Autodesk Fusion 360 part; units mm, degrees
(part 6 of 7)
  spline S1643 degree 3 poles (-40.457, 35.67) (-40.4097, 35.6808) (-40.3979, 35.7829) (-40.4495, 35.7797) knots 0 0 0 0 1 1 1 1
  spline S1644 degree 3 poles (-40.4495, 35.7797) (-40.501, 35.7764) (-40.5386, 35.7506) (-40.5773, 35.742) knots 0 0 0 0 1 1 1 1
  spline S1645 degree 3 poles (-40.5773, 35.742) (-40.6235, 35.7334) (-40.674, 35.626) (-40.6096, 35.6302) knots 0 0 0 0 1 1 1 1
  spline S1646 degree 3 poles (-40.5999, 35.2714) (-40.5451, 35.2736) (-40.4989, 35.2983) (-40.457, 35.3068) knots 0 0 0 0 1 1 1 1
  spline S1647 degree 3 poles (-40.457, 35.3068) (-40.414, 35.3176) (-40.4044, 35.4165) (-40.4516, 35.4121) knots 0 0 0 0 1 1 1 1
  spline S1648 degree 3 poles (-40.4516, 35.4121) (-40.4978, 35.4079) (-40.5365, 35.3863) (-40.572, 35.3788) knots 0 0 0 0 1 1 1 1
  spline S1649 degree 3 poles (-40.572, 35.3788) (-40.616, 35.3702) (-40.66, 35.2692) (-40.5999, 35.2714) knots 0 0 0 0 1 1 1 1
  spline S1650 degree 3 poles (-40.5784, 34.8684) (-40.5279, 34.8706) (-40.4828, 34.891) (-40.4441, 34.8996) knots 0 0 0 0 1 1 1 1
  spline S1651 degree 3 poles (-40.4441, 34.8996) (-40.4065, 34.9082) (-40.3958, 35.0006) (-40.4398, 34.9984) knots 0 0 0 0 1 1 1 1
  spline S1652 degree 3 poles (-40.4398, 34.9984) (-40.4839, 34.9941) (-40.5204, 34.9758) (-40.5526, 34.9694) knots 0 0 0 0 1 1 1 1
  spline S1653 degree 3 poles (-40.5526, 34.9694) (-40.5945, 34.963) (-40.6353, 34.8662) (-40.5784, 34.8684) knots 0 0 0 0 1 1 1 1
  spline S1654 degree 3 poles (-40.5118, 34.5664) (-40.4667, 34.5664) (-40.4216, 34.5857) (-40.3872, 34.5932) knots 0 0 0 0 1 1 1 1
  spline S1655 degree 3 poles (-40.3872, 34.5932) (-40.3528, 34.6018) (-40.3431, 34.6835) (-40.384, 34.6835) knots 0 0 0 0 1 1 1 1
  spline S1656 degree 3 poles (-40.384, 34.6835) (-40.4248, 34.6815) (-40.4592, 34.6643) (-40.4903, 34.6588) knots 0 0 0 0 1 1 1 1
  spline S1657 degree 3 poles (-40.4903, 34.6588) (-40.5301, 34.6546) (-40.5633, 34.5644) (-40.5118, 34.5664) knots 0 0 0 0 1 1 1 1
  spline S1658 degree 3 poles (-40.457, 34.1968) (-40.4162, 34.199) (-40.3711, 34.214) (-40.341, 34.2193) knots 0 0 0 0 1 1 1 1
  spline S1659 degree 3 poles (-40.341, 34.2193) (-40.3109, 34.2258) (-40.3023, 34.3009) (-40.3388, 34.3009) knots 0 0 0 0 1 1 1 1
  spline S1660 degree 3 poles (-40.3388, 34.3009) (-40.3764, 34.3009) (-40.4097, 34.2881) (-40.4377, 34.2817) knots 0 0 0 0 1 1 1 1
  spline S1661 degree 3 poles (-40.4377, 34.2817) (-40.4753, 34.2784) (-40.5032, 34.1924) (-40.457, 34.1968) knots 0 0 0 0 1 1 1 1
  spline S1662 degree 3 poles (-40.4022, 33.869) (-40.3646, 33.8712) (-40.3216, 33.8862) (-40.2948, 33.8906) knots 0 0 0 0 1 1 1 1
  spline S1663 degree 3 poles (-40.2948, 33.8906) (-40.269, 33.8948) (-40.2615, 33.9657) (-40.2948, 33.9679) knots 0 0 0 0 1 1 1 1
  spline S1664 degree 3 poles (-40.2948, 33.9679) (-40.3281, 33.97) (-40.3603, 33.9549) (-40.385, 33.9507) knots 0 0 0 0 1 1 1 1
  spline S1665 degree 3 poles (-40.385, 33.9507) (-40.4216, 33.9485) (-40.4441, 33.8668) (-40.4022, 33.869) knots 0 0 0 0 1 1 1 1
  spline S1666 degree 3 poles (-39.9478, 33.6702) (-39.9188, 33.6702) (-39.8747, 33.6788) (-39.8543, 33.681) knots 0 0 0 0 1 1 1 1
  spline S1667 degree 3 poles (-39.8543, 33.681) (-39.8339, 33.6852) (-39.8275, 33.7464) (-39.8565, 33.7475) knots 0 0 0 0 1 1 1 1
  spline S1668 degree 3 poles (-39.8565, 33.7475) (-39.8844, 33.7519) (-39.9156, 33.7411) (-39.936, 33.7411) knots 0 0 0 0 1 1 1 1
  spline S1669 degree 3 poles (-39.936, 33.7411) (-39.9682, 33.7389) (-39.9843, 33.6659) (-39.9478, 33.6702) knots 0 0 0 0 1 1 1 1
  spline S1670 degree 3 poles (-40.992, 35.1521) (-40.961, 35.1546) (-40.9301, 35.159) (-40.8996, 35.1649) knots 0 0 0 0 1 1 1 1
  spline S1671 degree 3 poles (-40.8996, 35.1649) (-40.8781, 35.1693) (-40.8717, 35.2305) (-40.9007, 35.2338) knots 0 0 0 0 1 1 1 1
  spline S1672 degree 3 poles (-40.9007, 35.2338) (-40.9286, 35.2359) (-40.9587, 35.2274) (-40.9802, 35.2252) knots 0 0 0 0 1 1 1 1
  spline S1673 degree 3 poles (-40.9802, 35.2252) (-41.0124, 35.223) (-41.0285, 35.1499) (-40.992, 35.1521) knots 0 0 0 0 1 1 1 1
  spline S1674 degree 3 poles (-39.4998, 33.7519) (-39.4611, 33.7583) (-39.387, 33.7605) (-39.3612, 33.7647) knots 0 0 0 0 1 1 1 1
  spline S1675 degree 3 poles (-39.3612, 33.7647) (-39.3354, 33.7691) (-39.3279, 33.855) (-39.3677, 33.8637) knots 0 0 0 0 1 1 1 1
  spline S1676 degree 3 poles (-39.3677, 33.8637) (-39.4074, 33.8743) (-39.4579, 33.8615) (-39.488, 33.8615) knots 0 0 0 0 1 1 1 1
  spline S1677 degree 3 poles (-39.488, 33.8615) (-39.5395, 33.8604) (-39.5514, 33.7455) (-39.4998, 33.7519) knots 0 0 0 0 1 1 1 1
  spline S1678 degree 3 poles (-39.4772, 33.4499) (-39.4407, 33.4543) (-39.3709, 33.4563) (-39.3462, 33.4607) knots 0 0 0 0 1 1 1 1
  spline S1679 degree 3 poles (-39.3462, 33.4607) (-39.3215, 33.4649) (-39.3139, 33.5466) (-39.3515, 33.5552) knots 0 0 0 0 1 1 1 1
  spline S1680 degree 3 poles (-39.3515, 33.5552) (-39.3891, 33.5659) (-39.4375, 33.5552) (-39.4665, 33.5552) knots 0 0 0 0 1 1 1 1
  spline S1681 degree 3 poles (-39.4665, 33.5552) (-39.5159, 33.5542) (-39.5266, 33.4435) (-39.4772, 33.4499) knots 0 0 0 0 1 1 1 1
  line L717 (-39.4289, 33.0889) -> (-39.3032, 33.0975)
  spline S1682 degree 3 poles (-39.3032, 33.0975) (-39.2796, 33.1017) (-39.272, 33.1792) (-39.3086, 33.1877) knots 0 0 0 0 1 1 1 1
  spline S1683 degree 3 poles (-39.3086, 33.1877) (-39.3451, 33.1985) (-39.3902, 33.1877) (-39.4171, 33.1877) knots 0 0 0 0 1 1 1 1
  spline S1684 degree 3 poles (-39.4171, 33.1877) (-39.4643, 33.1877) (-39.4751, 33.0823) (-39.4289, 33.0889) knots 0 0 0 0 1 1 1 1
  spline S1685 degree 3 poles (-39.373, 32.7299) (-39.3397, 32.7321) (-39.2763, 32.7363) (-39.2538, 32.7407) knots 0 0 0 0 1 1 1 1
  spline S1686 degree 3 poles (-39.2538, 32.7407) (-39.2323, 32.7429) (-39.2248, 32.818) (-39.2591, 32.8245) knots 0 0 0 0 1 1 1 1
  spline S1687 degree 3 poles (-39.2591, 32.8245) (-39.2946, 32.8353) (-39.3365, 32.8245) (-39.3623, 32.8245) knots 0 0 0 0 1 1 1 1
  spline S1688 degree 3 poles (-39.3623, 32.8245) (-39.4074, 32.8245) (-39.4171, 32.7257) (-39.373, 32.7299) knots 0 0 0 0 1 1 1 1
  spline S1689 degree 3 poles (-39.2828, 32.3893) (-39.2516, 32.3936) (-39.1915, 32.3979) (-39.17, 32.4) knots 0 0 0 0 1 1 1 1
  spline S1690 degree 3 poles (-39.17, 32.4) (-39.1496, 32.4043) (-39.1431, 32.4731) (-39.1754, 32.4796) knots 0 0 0 0 1 1 1 1
  spline S1691 degree 3 poles (-39.1754, 32.4796) (-39.2065, 32.4903) (-39.2484, 32.4796) (-39.2731, 32.4796) knots 0 0 0 0 1 1 1 1
  spline S1692 degree 3 poles (-39.2731, 32.4796) (-39.315, 32.4796) (-39.3247, 32.385) (-39.2828, 32.3893) knots 0 0 0 0 1 1 1 1
  line L718 (-39.2258, 32.0186) -> (-39.1206, 32.0271)
  spline S1693 degree 3 poles (-39.1206, 32.0271) (-39.1012, 32.0315) (-39.0948, 32.0959) (-39.1249, 32.1024) knots 0 0 0 0 1 1 1 1
  spline S1694 degree 3 poles (-39.1249, 32.1024) (-39.1549, 32.111) (-39.1936, 32.1024) (-39.2162, 32.1024) knots 0 0 0 0 1 1 1 1
  spline S1695 degree 3 poles (-39.2162, 32.1024) (-39.2559, 32.1024) (-39.2656, 32.0143) (-39.2258, 32.0186) knots 0 0 0 0 1 1 1 1
  line L719 (-39.1216, 31.7037) -> (-39.0239, 31.7101)
  spline S1696 degree 3 poles (-39.0239, 31.7101) (-39.0045, 31.7144) (-39.0002, 31.7757) (-39.0271, 31.7832) knots 0 0 0 0 1 1 1 1
  spline S1697 degree 3 poles (-39.0271, 31.7832) (-39.0561, 31.7897) (-39.0916, 31.7811) (-39.1141, 31.7811) knots 0 0 0 0 1 1 1 1
  spline S1698 degree 3 poles (-39.1141, 31.7811) (-39.1506, 31.7811) (-39.1592, 31.6973) (-39.1216, 31.7037) knots 0 0 0 0 1 1 1 1
  spline S1699 degree 3 poles (-39.0325, 31.3899) (-39.0067, 31.3931) (-38.9573, 31.3953) (-38.9401, 31.3974) knots 0 0 0 0 1 1 1 1
  spline S1700 degree 3 poles (-38.9401, 31.3974) (-38.9229, 31.4007) (-38.9175, 31.4598) (-38.9444, 31.4662) knots 0 0 0 0 1 1 1 1
  spline S1701 degree 3 poles (-38.9444, 31.4662) (-38.9712, 31.4727) (-39.0045, 31.4641) (-39.025, 31.4641) knots 0 0 0 0 1 1 1 1
  spline S1702 degree 3 poles (-39.025, 31.4641) (-39.0593, 31.4641) (-39.0668, 31.3867) (-39.0325, 31.3899) knots 0 0 0 0 1 1 1 1
  spline S1703 degree 3 poles (-39.431, 31.2846) (-39.4074, 31.2889) (-39.358, 31.2911) (-39.3397, 31.2932) knots 0 0 0 0 1 1 1 1
  spline S1704 degree 3 poles (-39.3397, 31.2932) (-39.3236, 31.2964) (-39.3172, 31.3534) (-39.344, 31.3598) knots 0 0 0 0 1 1 1 1
  spline S1705 degree 3 poles (-39.344, 31.3598) (-39.3709, 31.3663) (-39.4042, 31.3577) (-39.4246, 31.3577) knots 0 0 0 0 1 1 1 1
  spline S1706 degree 3 poles (-39.4246, 31.3577) (-39.4579, 31.3577) (-39.4665, 31.2803) (-39.431, 31.2846) knots 0 0 0 0 1 1 1 1
  spline S1707 degree 3 poles (-38.925, 31.0976) (-38.9014, 31.1009) (-38.8552, 31.103) (-38.8402, 31.1051) knots 0 0 0 0 1 1 1 1
  spline S1708 degree 3 poles (-38.8402, 31.1051) (-38.8241, 31.1084) (-38.8187, 31.161) (-38.8434, 31.1675) knots 0 0 0 0 1 1 1 1
  spline S1709 degree 3 poles (-38.8434, 31.1675) (-38.8681, 31.1718) (-38.8993, 31.1643) (-38.9175, 31.1643) knots 0 0 0 0 1 1 1 1
  spline S1710 degree 3 poles (-38.9175, 31.1643) (-38.9498, 31.1643) (-38.9573, 31.0933) (-38.925, 31.0976) knots 0 0 0 0 1 1 1 1
  line L720 (-39.5181, 31.6317) -> (-39.4321, 31.6381)
  spline S1711 degree 3 poles (-39.4321, 31.6381) (-39.4171, 31.6424) (-39.4117, 31.6951) (-39.4364, 31.7015) knots 0 0 0 0 1 1 1 1
  spline S1712 degree 3 poles (-39.4364, 31.7015) (-39.4611, 31.708) (-39.4923, 31.6994) (-39.5116, 31.6994) knots 0 0 0 0 1 1 1 1
  spline S1713 degree 3 poles (-39.5116, 31.6994) (-39.5428, 31.6994) (-39.5503, 31.6274) (-39.5181, 31.6317) knots 0 0 0 0 1 1 1 1
  spline S1714 degree 3 poles (-39.2946, 30.9934) (-39.272, 30.9955) (-39.2258, 30.9977) (-39.2086, 31.0009) knots 0 0 0 0 1 1 1 1
  spline S1715 degree 3 poles (-39.2086, 31.0009) (-39.1936, 31.0031) (-39.1882, 31.0579) (-39.213, 31.0643) knots 0 0 0 0 1 1 1 1
  spline S1716 degree 3 poles (-39.213, 31.0643) (-39.2377, 31.0708) (-39.2688, 31.0632) (-39.2871, 31.0632) knots 0 0 0 0 1 1 1 1
  spline S1717 degree 3 poles (-39.2871, 31.0632) (-39.3193, 31.0622) (-39.3268, 30.9891) (-39.2946, 30.9934) knots 0 0 0 0 1 1 1 1
  line L721 (-38.823, 30.7892) -> (-38.7446, 30.7967)
  spline S1718 degree 3 poles (-38.7446, 30.7967) (-38.7295, 30.7989) (-38.7241, 30.8483) (-38.7478, 30.8537) knots 0 0 0 0 1 1 1 1
  spline S1719 degree 3 poles (-38.7478, 30.8537) (-38.7703, 30.8591) (-38.7983, 30.8526) (-38.8165, 30.8526) knots 0 0 0 0 1 1 1 1
  spline S1720 degree 3 poles (-38.8165, 30.8526) (-38.8455, 30.8515) (-38.852, 30.7849) (-38.823, 30.7892) knots 0 0 0 0 1 1 1 1
  line L722 (-39.575, 32.0014) -> (-39.4966, 32.0078)
  spline S1721 degree 3 poles (-39.4966, 32.0078) (-39.4815, 32.01) (-39.4772, 32.0583) (-39.4998, 32.0648) knots 0 0 0 0 1 1 1 1
  spline S1722 degree 3 poles (-39.4998, 32.0648) (-39.5224, 32.0691) (-39.5514, 32.0626) (-39.5685, 32.0626) knots 0 0 0 0 1 1 1 1
  spline S1723 degree 3 poles (-39.5685, 32.0626) (-39.5986, 32.0626) (-39.6051, 31.9971) (-39.575, 32.0014) knots 0 0 0 0 1 1 1 1
  spline S1724 degree 3 poles (-40.8104, 34.1376) (-40.7879, 34.142) (-40.746, 34.1442) (-40.7309, 34.1462) knots 0 0 0 0 1 1 1 1
  spline S1725 degree 3 poles (-40.7309, 34.1462) (-40.7159, 34.1484) (-40.7116, 34.199) (-40.7342, 34.2054) knots 0 0 0 0 1 1 1 1
  spline S1726 degree 3 poles (-40.7342, 34.2054) (-40.7578, 34.2096) (-40.7857, 34.2032) (-40.8029, 34.2032) knots 0 0 0 0 1 1 1 1
  spline S1727 degree 3 poles (-40.8029, 34.2032) (-40.833, 34.2032) (-40.8395, 34.1356) (-40.8104, 34.1376) knots 0 0 0 0 1 1 1 1
  line L723 (-39.9113, 33.322) -> (-39.8317, 33.3284)
  spline S1728 degree 3 poles (-39.8317, 33.3284) (-39.8178, 33.3306) (-39.8124, 33.379) (-39.835, 33.3854) knots 0 0 0 0 1 1 1 1
  spline S1729 degree 3 poles (-39.835, 33.3854) (-39.8586, 33.3918) (-39.8865, 33.3854) (-39.9048, 33.3854) knots 0 0 0 0 1 1 1 1
  spline S1730 degree 3 poles (-39.9048, 33.3854) (-39.9338, 33.3843) (-39.9413, 33.3178) (-39.9113, 33.322) knots 0 0 0 0 1 1 1 1
  line L724 (-40.9415, 34.8094) -> (-40.8609, 34.8158)
  spline S1731 degree 3 poles (-40.8609, 34.8158) (-40.847, 34.8179) (-40.8427, 34.8684) (-40.8652, 34.8748) knots 0 0 0 0 1 1 1 1
  spline S1732 degree 3 poles (-40.8652, 34.8748) (-40.8878, 34.8791) (-40.9168, 34.8727) (-40.934, 34.8727) knots 0 0 0 0 1 1 1 1
  spline S1733 degree 3 poles (-40.934, 34.8727) (-40.9641, 34.8727) (-40.9705, 34.805) (-40.9415, 34.8094) knots 0 0 0 0 1 1 1 1
  line L725 (-39.2054, 30.7033) -> (-39.127, 30.7097)
  spline S1734 degree 3 poles (-39.127, 30.7097) (-39.113, 30.7119) (-39.1077, 30.7602) (-39.1302, 30.7666) knots 0 0 0 0 1 1 1 1
  spline S1735 degree 3 poles (-39.1302, 30.7666) (-39.1539, 30.772) (-39.1818, 30.7656) (-39.2001, 30.7656) knots 0 0 0 0 1 1 1 1
  spline S1736 degree 3 poles (-39.2001, 30.7656) (-39.2291, 30.7645) (-39.2366, 30.699) (-39.2054, 30.7033) knots 0 0 0 0 1 1 1 1
  spline S1737 degree 3 poles (-40.6729, 33.4768) (-40.6504, 33.4811) (-40.6085, 33.4832) (-40.5924, 33.4854) knots 0 0 0 0 1 1 1 1
  spline S1738 degree 3 poles (-40.5924, 33.4854) (-40.5784, 33.4875) (-40.5741, 33.538) (-40.5967, 33.5424) knots 0 0 0 0 1 1 1 1
  spline S1739 degree 3 poles (-40.5967, 33.5424) (-40.6192, 33.5466) (-40.6482, 33.5402) (-40.6654, 33.5402) knots 0 0 0 0 1 1 1 1
  spline S1740 degree 3 poles (-40.6654, 33.5402) (-40.6955, 33.5402) (-40.7019, 33.4746) (-40.6729, 33.4768) knots 0 0 0 0 1 1 1 1
  line L726 (-40.5483, 32.8288) -> (-40.471, 32.8353)
  spline S1741 degree 3 poles (-40.471, 32.8353) (-40.457, 32.8373) (-40.4505, 32.8879) (-40.4731, 32.8943) knots 0 0 0 0 1 1 1 1
  spline S1742 degree 3 poles (-40.4731, 32.8943) (-40.4968, 32.9007) (-40.5247, 32.8922) (-40.5429, 32.8922) knots 0 0 0 0 1 1 1 1
  spline S1743 degree 3 poles (-40.5429, 32.8922) (-40.572, 32.8911) (-40.5795, 32.8245) (-40.5483, 32.8288) knots 0 0 0 0 1 1 1 1
  line L727 (-38.7123, 30.4679) -> (-38.6414, 30.4744)
  spline S1744 degree 3 poles (-38.6414, 30.4744) (-38.6275, 30.4765) (-38.6232, 30.5217) (-38.6446, 30.527) knots 0 0 0 0 1 1 1 1
  spline S1745 degree 3 poles (-38.6446, 30.527) (-38.6651, 30.5324) (-38.6919, 30.5259) (-38.708, 30.5259) knots 0 0 0 0 1 1 1 1
  spline S1746 degree 3 poles (-38.708, 30.5259) (-38.7338, 30.5259) (-38.7403, 30.4647) (-38.7123, 30.4679) knots 0 0 0 0 1 1 1 1
  spline S1747 degree 3 poles (-40.0047, 36.2202) (-39.966, 36.2309) (-39.9424, 36.2954) (-39.9596, 36.2954) knots 0 0 0 0 1 1 1 1
  spline S1748 degree 3 poles (-39.9596, 36.2954) (-39.9725, 36.2976) (-40.0079, 36.3223) (-40.0552, 36.3126) knots 0 0 0 0 1 1 1 1
  spline S1749 degree 3 poles (-40.0552, 36.3126) (-40.0982, 36.304) (-40.1369, 36.2375) (-40.1089, 36.2353) knots 0 0 0 0 1 1 1 1
  spline S1750 degree 3 poles (-40.1089, 36.2353) (-40.0982, 36.2287) (-40.0552, 36.201) (-40.0047, 36.2202) knots 0 0 0 0 1 1 1 1
  spline S1751 degree 3 poles (-39.9306, 36.6855) (-39.908, 36.6984) (-39.8758, 36.7048) (-39.8489, 36.7145) knots 0 0 0 0 1 1 1 1
  spline S1752 degree 3 poles (-39.8489, 36.7145) (-39.8167, 36.7253) (-39.8135, 36.8048) (-39.864, 36.7962) knots 0 0 0 0 1 1 1 1
  spline S1753 degree 3 poles (-39.864, 36.7962) (-39.8951, 36.7898) (-39.9102, 36.7746) (-39.9306, 36.7693) knots 0 0 0 0 1 1 1 1
  spline S1754 degree 3 poles (-39.9306, 36.7693) (-39.98, 36.7575) (-39.9768, 36.6672) (-39.9306, 36.6855) knots 0 0 0 0 1 1 1 1
  spline S1755 degree 3 poles (-41.7268, 26.8315) (-41.7526, 26.8981) (-41.7537, 26.8841) (-41.7537, 26.9336) knots 0 0 0 0 1 1 1 1
  spline S1756 degree 3 poles (-41.7537, 26.9336) (-41.7537, 26.9841) (-41.7064, 27.0228) (-41.6785, 26.9422) knots 0 0 0 0 1 1 1 1
  spline S1757 degree 2 poles (-41.6785, 26.9422) (-41.6581, 26.882) (-41.6559, 26.8347) knots 0 0 0 1 1 1
  spline S1758 degree 2 poles (-41.6559, 26.8347) (-41.7204, 26.8143) (-41.7268, 26.8315) knots 0 0 0 1 1 1
  spline S1759 degree 3 poles (-41.9621, 26.7133) (-41.9868, 26.7799) (-41.989, 26.7659) (-41.989, 26.8164) knots 0 0 0 0 1 1 1 1
  spline S1760 degree 3 poles (-41.989, 26.8164) (-41.989, 26.8669) (-41.9417, 26.9056) (-41.9138, 26.825) knots 0 0 0 0 1 1 1 1
  spline S1761 degree 2 poles (-41.9138, 26.825) (-41.8912, 26.7638) (-41.8901, 26.7176) knots 0 0 0 1 1 1
  spline S1762 degree 2 poles (-41.8901, 26.7176) (-41.9557, 26.6972) (-41.9621, 26.7133) knots 0 0 0 1 1 1
  spline S1763 degree 3 poles (-41.599, 26.4769) (-41.6226, 26.5435) (-41.6259, 26.5284) (-41.6259, 26.579) knots 0 0 0 0 1 1 1 1
  spline S1764 degree 3 poles (-41.6259, 26.579) (-41.6259, 26.6295) (-41.5786, 26.6681) (-41.5506, 26.5876) knots 0 0 0 0 1 1 1 1
  spline S1765 degree 2 poles (-41.5506, 26.5876) (-41.5302, 26.5274) (-41.5281, 26.4812) knots 0 0 0 1 1 1
  spline S1766 degree 2 poles (-41.5281, 26.4812) (-41.5925, 26.4597) (-41.599, 26.4769) knots 0 0 0 1 1 1
  spline S1767 degree 3 poles (-41.7999, 27.2323) (-41.8257, 27.2989) (-41.8278, 27.285) (-41.8278, 27.3344) knots 0 0 0 0 1 1 1 1
  spline S1768 degree 3 poles (-41.8278, 27.3344) (-41.8278, 27.3849) (-41.7795, 27.4236) (-41.7526, 27.343) knots 0 0 0 0 1 1 1 1
  spline S1769 degree 3 poles (-41.7526, 27.343) (-41.74, 27.3088) (-41.7324, 27.273) (-41.73, 27.2366) knots 0 0 0 0 1 1 1 1
  spline S1770 degree 2 poles (-41.73, 27.2366) (-41.7945, 27.2151) (-41.7999, 27.2323) knots 0 0 0 1 1 1
  spline S1771 degree 3 poles (-40.2669, 28.5272) (-40.2916, 28.5938) (-40.2937, 28.5799) (-40.2937, 28.6304) knots 0 0 0 0 1 1 1 1
  spline S1772 degree 3 poles (-40.2937, 28.6304) (-40.2937, 28.6798) (-40.2464, 28.7195) (-40.2185, 28.6379) knots 0 0 0 0 1 1 1 1
  spline S1773 degree 2 poles (-40.2185, 28.6379) (-40.197, 28.5777) (-40.1949, 28.5315) knots 0 0 0 1 1 1
  spline S1774 degree 2 poles (-40.1949, 28.5315) (-40.2604, 28.51) (-40.2669, 28.5272) knots 0 0 0 1 1 1
  spline S1775 degree 3 poles (-37.1342, 28.4079) (-37.1589, 28.4745) (-37.161, 28.4595) (-37.161, 28.5111) knots 0 0 0 0 1 1 1 1
  spline S1776 degree 3 poles (-37.161, 28.5111) (-37.161, 28.5616) (-37.1148, 28.6003) (-37.0858, 28.5197) knots 0 0 0 0 1 1 1 1
  spline S1777 degree 2 poles (-37.0858, 28.5197) (-37.0643, 28.4584) (-37.0622, 28.4122) knots 0 0 0 1 1 1
  spline S1778 degree 2 poles (-37.0622, 28.4122) (-37.1277, 28.3907) (-37.1342, 28.4079) knots 0 0 0 1 1 1
  spline S1779 degree 3 poles (-41.6871, 27.4558) (-41.6892, 27.5085) (-41.6387, 27.5525) (-41.6097, 27.4698) knots 0 0 0 0 1 1 1 1
  spline S1780 degree 3 poles (-41.6097, 27.4698) (-41.5861, 27.4053) (-41.585, 27.3602) (-41.5839, 27.3559) knots 0 0 0 0 1 1 1 1
  spline S1781 degree 3 poles (-41.5839, 27.3559) (-41.5818, 27.3527) (-41.6506, 27.329) (-41.6591, 27.3484) knots 0 0 0 0 1 1 1 1
  spline S1782 degree 3 poles (-41.6591, 27.3484) (-41.6839, 27.415) (-41.686, 27.4053) (-41.6871, 27.4558) knots 0 0 0 0 1 1 1 1
  spline S1783 degree 3 poles (-36.5229, 29.3321) (-36.525, 29.3858) (-36.4745, 29.4288) (-36.4455, 29.346) knots 0 0 0 0 1 1 1 1
  spline S1784 degree 3 poles (-36.4455, 29.346) (-36.423, 29.2816) (-36.4219, 29.2375) (-36.4198, 29.2343) knots 0 0 0 0 1 1 1 1
  spline S1785 degree 3 poles (-36.4198, 29.2343) (-36.4187, 29.2311) (-36.4864, 29.2063) (-36.495, 29.2268) knots 0 0 0 0 1 1 1 1
  spline S1786 degree 3 poles (-36.495, 29.2268) (-36.5197, 29.2923) (-36.5218, 29.2816) (-36.5229, 29.3321) knots 0 0 0 0 1 1 1 1
  spline S1787 degree 3 poles (-36.6411, 29.7694) (-36.6432, 29.8232) (-36.5916, 29.8651) (-36.5626, 29.7823) knots 0 0 0 0 1 1 1 1
  spline S1788 degree 3 poles (-36.5626, 29.7823) (-36.549, 29.7462) (-36.541, 29.7081) (-36.539, 29.6695) knots 0 0 0 0 1 1 1 1
  spline S1789 degree 3 poles (-36.539, 29.6695) (-36.5369, 29.6663) (-36.6045, 29.6426) (-36.6121, 29.662) knots 0 0 0 0 1 1 1 1
  spline S1790 degree 3 poles (-36.6121, 29.662) (-36.6378, 29.7297) (-36.64, 29.7189) (-36.6411, 29.7694) knots 0 0 0 0 1 1 1 1
  spline S1791 degree 3 poles (-41.4916, 27.5697) (-41.4948, 27.6256) (-41.4421, 27.6729) (-41.4121, 27.588) knots 0 0 0 0 1 1 1 1
  spline S1792 degree 3 poles (-41.4121, 27.588) (-41.3873, 27.5214) (-41.3873, 27.4762) (-41.3841, 27.4698) knots 0 0 0 0 1 1 1 1
  spline S1793 degree 3 poles (-41.3841, 27.4698) (-41.3798, 27.4612) (-41.4529, 27.4354) (-41.4615, 27.458) knots 0 0 0 0 1 1 1 1
  spline S1794 degree 3 poles (-41.4615, 27.458) (-41.4873, 27.5246) (-41.4894, 27.5192) (-41.4916, 27.5697) knots 0 0 0 0 1 1 1 1
  spline S1795 degree 3 poles (-41.2735, 27.6707) (-41.2788, 27.7288) (-41.223, 27.7814) (-41.1908, 27.6944) knots 0 0 0 0 1 1 1 1
  spline S1796 degree 3 poles (-41.1908, 27.6944) (-41.166, 27.6245) (-41.1671, 27.5805) (-41.1607, 27.5687) knots 0 0 0 0 1 1 1 1
  spline S1797 degree 3 poles (-41.1607, 27.5687) (-41.1553, 27.5579) (-41.2316, 27.5289) (-41.2423, 27.5547) knots 0 0 0 0 1 1 1 1
  spline S1798 degree 3 poles (-41.2423, 27.5547) (-41.2692, 27.6213) (-41.2703, 27.6202) (-41.2735, 27.6707) knots 0 0 0 0 1 1 1 1
  spline S1799 degree 3 poles (-36.7753, 29.2654) (-36.7807, 29.3245) (-36.7238, 29.3761) (-36.6926, 29.2891) knots 0 0 0 0 1 1 1 1
  spline S1800 degree 3 poles (-36.6926, 29.2891) (-36.6669, 29.2192) (-36.669, 29.1752) (-36.6615, 29.1634) knots 0 0 0 0 1 1 1 1
  spline S1801 degree 3 poles (-36.6615, 29.1634) (-36.6561, 29.1526) (-36.7334, 29.1236) (-36.7431, 29.1483) knots 0 0 0 0 1 1 1 1
  spline S1802 degree 3 poles (-36.7431, 29.1483) (-36.77, 29.216) (-36.7721, 29.2149) (-36.7753, 29.2654) knots 0 0 0 0 1 1 1 1
  spline S1803 degree 3 poles (-41.0393, 27.7718) (-41.0457, 27.833) (-40.9866, 27.89) (-40.9533, 27.8008) knots 0 0 0 0 1 1 1 1
  spline S1804 degree 3 poles (-40.9533, 27.8008) (-40.9265, 27.7266) (-40.9286, 27.6836) (-40.9211, 27.6686) knots 0 0 0 0 1 1 1 1
  spline S1805 degree 3 poles (-40.9211, 27.6686) (-40.9136, 27.6536) (-40.9941, 27.6224) (-41.006, 27.6503) knots 0 0 0 0 1 1 1 1
  spline S1806 degree 3 poles (-41.006, 27.6503) (-41.026, 27.6878) (-41.0374, 27.7293) (-41.0393, 27.7718) knots 0 0 0 0 1 1 1 1
  spline S1807 degree 3 poles (-37.3125, 29.1322) (-37.32, 29.1934) (-37.2599, 29.2493) (-37.2276, 29.1601) knots 0 0 0 0 1 1 1 1
  spline S1808 degree 3 poles (-37.2276, 29.1601) (-37.1997, 29.0871) (-37.2018, 29.043) (-37.1943, 29.029) knots 0 0 0 0 1 1 1 1
  spline S1809 degree 3 poles (-37.1943, 29.029) (-37.1879, 29.0129) (-37.2674, 28.9839) (-37.2813, 29.0108) knots 0 0 0 0 1 1 1 1
  spline S1810 degree 3 poles (-37.2813, 29.0108) (-37.2999, 29.0487) (-37.3105, 29.09) (-37.3125, 29.1322) knots 0 0 0 0 1 1 1 1
  spline S1811 degree 3 poles (-37.7659, 29.6007) (-37.7723, 29.662) (-37.7132, 29.72) (-37.681, 29.6308) knots 0 0 0 0 1 1 1 1
  spline S1812 degree 3 poles (-37.681, 29.6308) (-37.6531, 29.5567) (-37.6552, 29.5137) (-37.6477, 29.4986) knots 0 0 0 0 1 1 1 1
  spline S1813 degree 3 poles (-37.6477, 29.4986) (-37.6402, 29.4836) (-37.7207, 29.4524) (-37.7326, 29.4804) knots 0 0 0 0 1 1 1 1
  spline S1814 degree 3 poles (-37.7326, 29.4804) (-37.7605, 29.5481) (-37.7616, 29.5502) (-37.7659, 29.6007) knots 0 0 0 0 1 1 1 1
  spline S1815 degree 3 poles (-38.0667, 29.5384) (-38.0742, 29.5986) (-38.014, 29.6544) (-37.9818, 29.5653) knots 0 0 0 0 1 1 1 1
  spline S1816 degree 3 poles (-37.9818, 29.5653) (-37.9539, 29.4922) (-37.956, 29.4492) (-37.9496, 29.4342) knots 0 0 0 0 1 1 1 1
  spline S1817 degree 3 poles (-37.9496, 29.4342) (-37.941, 29.4191) (-38.0215, 29.3879) (-38.0344, 29.4148) knots 0 0 0 0 1 1 1 1
  spline S1818 degree 3 poles (-38.0344, 29.4148) (-38.0536, 29.4534) (-38.0645, 29.4954) (-38.0667, 29.5384) knots 0 0 0 0 1 1 1 1
  spline S1819 degree 3 poles (-39.8479, 28.884) (-39.8554, 28.9452) (-39.7952, 29.0022) (-39.763, 28.913) knots 0 0 0 0 1 1 1 1
  spline S1820 degree 3 poles (-39.763, 28.913) (-39.7361, 28.8399) (-39.7383, 28.7958) (-39.7308, 28.7819) knots 0 0 0 0 1 1 1 1
  spline S1821 degree 3 poles (-39.7308, 28.7819) (-39.7222, 28.7668) (-39.8027, 28.7357) (-39.8156, 28.7625) knots 0 0 0 0 1 1 1 1
  spline S1822 degree 3 poles (-39.8156, 28.7625) (-39.8347, 28.8003) (-39.8457, 28.8417) (-39.8479, 28.884) knots 0 0 0 0 1 1 1 1
  spline S1823 degree 3 poles (-40.1003, 28.7496) (-40.1068, 28.8109) (-40.0477, 28.8678) (-40.0144, 28.7787) knots 0 0 0 0 1 1 1 1
  spline S1824 degree 3 poles (-40.0144, 28.7787) (-39.9875, 28.7056) (-39.9897, 28.6615) (-39.9821, 28.6475) knots 0 0 0 0 1 1 1 1
  spline S1825 degree 3 poles (-39.9821, 28.6475) (-39.9746, 28.6325) (-40.0531, 28.6013) (-40.067, 28.6293) knots 0 0 0 0 1 1 1 1
  spline S1826 degree 3 poles (-40.067, 28.6293) (-40.095, 28.6959) (-40.0949, 28.7002) (-40.1003, 28.7496) knots 0 0 0 0 1 1 1 1
  spline S1827 degree 3 poles (-37.161, 29.7522) (-37.1685, 29.8135) (-37.1095, 29.8704) (-37.0761, 29.7813) knots 0 0 0 0 1 1 1 1
  spline S1828 degree 3 poles (-37.0761, 29.7813) (-37.0493, 29.7082) (-37.0514, 29.6652) (-37.0439, 29.6491) knots 0 0 0 0 1 1 1 1
  spline S1829 degree 3 poles (-37.0439, 29.6491) (-37.0364, 29.6351) (-37.1159, 29.6029) (-37.1288, 29.6319) knots 0 0 0 0 1 1 1 1
  spline S1830 degree 3 poles (-37.1288, 29.6319) (-37.1557, 29.6985) (-37.1578, 29.7017) (-37.161, 29.7522) knots 0 0 0 0 1 1 1 1
  spline S1831 degree 3 poles (-40.8545, 27.8728) (-40.8631, 27.9351) (-40.8008, 27.9974) (-40.7664, 27.9061) knots 0 0 0 0 1 1 1 1
  spline S1832 degree 3 poles (-40.7664, 27.9061) (-40.7374, 27.8298) (-40.7406, 27.7868) (-40.7309, 27.7685) knots 0 0 0 0 1 1 1 1
  spline S1833 degree 3 poles (-40.7309, 27.7685) (-40.7224, 27.7492) (-40.8072, 27.7159) (-40.8201, 27.746) knots 0 0 0 0 1 1 1 1
  spline S1834 degree 3 poles (-40.8201, 27.746) (-40.8399, 27.7855) (-40.8516, 27.8286) (-40.8545, 27.8728) knots 0 0 0 0 1 1 1 1
  spline S1835 degree 3 poles (-40.602, 27.9727) (-40.6128, 28.0383) (-40.5472, 28.1049) (-40.5129, 28.0114) knots 0 0 0 0 1 1 1 1
  spline S1836 degree 3 poles (-40.5129, 28.0114) (-40.4817, 27.9319) (-40.486, 27.89) (-40.4753, 27.8685) knots 0 0 0 0 1 1 1 1
  spline S1837 degree 3 poles (-40.4753, 27.8685) (-40.4624, 27.8459) (-40.5515, 27.8094) (-40.5676, 27.8427) knots 0 0 0 0 1 1 1 1
  spline S1838 degree 3 poles (-40.5676, 27.8427) (-40.5872, 27.8835) (-40.5988, 27.9276) (-40.602, 27.9727) knots 0 0 0 0 1 1 1 1
  spline S1839 degree 3 poles (-37.624, 29.0355) (-37.6348, 29.101) (-37.5703, 29.1666) (-37.5349, 29.0742) knots 0 0 0 0 1 1 1 1
  spline S1840 degree 3 poles (-37.5349, 29.0742) (-37.5037, 28.9936) (-37.508, 28.9517) (-37.4973, 28.9302) knots 0 0 0 0 1 1 1 1
  spline S1841 degree 3 poles (-37.4973, 28.9302) (-37.4855, 28.9076) (-37.5736, 28.8711) (-37.5897, 28.9055) knots 0 0 0 0 1 1 1 1
  spline S1842 degree 3 poles (-37.5897, 28.9055) (-37.6092, 28.9462) (-37.6209, 28.9904) (-37.624, 29.0355) knots 0 0 0 0 1 1 1 1
  spline S1843 degree 3 poles (-37.4855, 29.6964) (-37.4962, 29.763) (-37.4317, 29.8285) (-37.3963, 29.735) knots 0 0 0 0 1 1 1 1
  spline S1844 degree 3 poles (-37.3963, 29.735) (-37.3662, 29.6555) (-37.3694, 29.6136) (-37.3587, 29.5921) knots 0 0 0 0 1 1 1 1
  spline S1845 degree 3 poles (-37.3587, 29.5921) (-37.3469, 29.5696) (-37.435, 29.533) (-37.4511, 29.5663) knots 0 0 0 0 1 1 1 1
  spline S1846 degree 3 poles (-37.4511, 29.5663) (-37.479, 29.634) (-37.4801, 29.6459) (-37.4855, 29.6964) knots 0 0 0 0 1 1 1 1
  spline S1847 degree 3 poles (-40.4173, 28.0565) (-40.4301, 28.1253) (-40.3625, 28.1962) (-40.3259, 28.1006) knots 0 0 0 0 1 1 1 1
  spline S1848 degree 3 poles (-40.3259, 28.1006) (-40.2937, 28.0178) (-40.2991, 27.977) (-40.2851, 27.9512) knots 0 0 0 0 1 1 1 1
  spline S1849 degree 3 poles (-40.2851, 27.9512) (-40.2733, 27.9243) (-40.3635, 27.8857) (-40.3818, 27.9222) knots 0 0 0 0 1 1 1 1
  spline S1850 degree 3 poles (-40.3818, 27.9222) (-40.4097, 27.9888) (-40.4108, 28.0071) (-40.4173, 28.0565) knots 0 0 0 0 1 1 1 1
  spline S1851 degree 3 poles (-37.8905, 28.9194) (-37.9034, 28.9871) (-37.8357, 29.058) (-37.7992, 28.9635) knots 0 0 0 0 1 1 1 1
  spline S1852 degree 3 poles (-37.7992, 28.9635) (-37.7669, 28.8807) (-37.7712, 28.8388) (-37.7594, 28.813) knots 0 0 0 0 1 1 1 1
  spline S1853 degree 3 poles (-37.7594, 28.813) (-37.7455, 28.7873) (-37.8378, 28.7486) (-37.855, 28.7851) knots 0 0 0 0 1 1 1 1
  spline S1854 degree 3 poles (-37.855, 28.7851) (-37.883, 28.8517) (-37.884, 28.8689) (-37.8905, 28.9194) knots 0 0 0 0 1 1 1 1
  spline S1855 degree 3 poles (-38.3535, 29.4503) (-38.3653, 29.519) (-38.2976, 29.59) (-38.2611, 29.4954) knots 0 0 0 0 1 1 1 1
  spline S1856 degree 3 poles (-38.2611, 29.4954) (-38.2289, 29.4127) (-38.2343, 29.3708) (-38.2203, 29.3428) knots 0 0 0 0 1 1 1 1
  spline S1857 degree 3 poles (-38.2203, 29.3428) (-38.2085, 29.317) (-38.2998, 29.2783) (-38.317, 29.3149) knots 0 0 0 0 1 1 1 1
  spline S1858 degree 3 poles (-38.317, 29.3149) (-38.3449, 29.3826) (-38.3471, 29.4008) (-38.3535, 29.4503) knots 0 0 0 0 1 1 1 1
  spline S1859 degree 3 poles (-38.5716, 29.3493) (-38.5834, 29.4191) (-38.5157, 29.489) (-38.4792, 29.3944) knots 0 0 0 0 1 1 1 1
  spline S1860 degree 3 poles (-38.4792, 29.3944) (-38.447, 29.3117) (-38.4523, 29.2697) (-38.4395, 29.2429) knots 0 0 0 0 1 1 1 1
  spline S1861 degree 3 poles (-38.4395, 29.2429) (-38.4266, 29.2171) (-38.5179, 29.1784) (-38.5351, 29.2149) knots 0 0 0 0 1 1 1 1
  spline S1862 degree 3 poles (-38.5351, 29.2149) (-38.563, 29.2816) (-38.5651, 29.2988) (-38.5716, 29.3493) knots 0 0 0 0 1 1 1 1
  spline S1863 degree 3 poles (-38.8402, 29.2321) (-38.852, 29.3009) (-38.7843, 29.3718) (-38.7478, 29.2773) knots 0 0 0 0 1 1 1 1
  spline S1864 degree 3 poles (-38.7478, 29.2773) (-38.7155, 29.1934) (-38.7209, 29.1526) (-38.708, 29.1257) knots 0 0 0 0 1 1 1 1
  spline S1865 degree 3 poles (-38.708, 29.1257) (-38.6951, 29.1) (-38.7865, 29.0613) (-38.8036, 29.0978) knots 0 0 0 0 1 1 1 1
  spline S1866 degree 3 poles (-38.8036, 29.0978) (-38.8316, 29.1644) (-38.8337, 29.1816) (-38.8402, 29.2321) knots 0 0 0 0 1 1 1 1
  spline S1867 degree 3 poles (-40.1659, 28.1575) (-40.1809, 28.2285) (-40.1089, 28.3037) (-40.0713, 28.207) knots 0 0 0 0 1 1 1 1
  spline S1868 degree 3 poles (-40.0713, 28.207) (-40.038, 28.121) (-40.0445, 28.0802) (-40.0294, 28.0512) knots 0 0 0 0 1 1 1 1
  spline S1869 degree 3 poles (-40.0294, 28.0512) (-40.0133, 28.0211) (-40.11, 27.9792) (-40.1283, 28.0178) knots 0 0 0 0 1 1 1 1
  spline S1870 degree 3 poles (-40.1283, 28.0178) (-40.1573, 28.0855) (-40.1583, 28.107) (-40.1659, 28.1575) knots 0 0 0 0 1 1 1 1
  spline S1871 degree 3 poles (-38.1279, 28.8464) (-38.1429, 28.9183) (-38.072, 28.9936) (-38.0344, 28.8969) knots 0 0 0 0 1 1 1 1
  spline S1872 degree 3 poles (-38.0344, 28.8969) (-38.0001, 28.8098) (-38.0065, 28.769) (-37.9915, 28.74) knots 0 0 0 0 1 1 1 1
  spline S1873 degree 3 poles (-37.9915, 28.74) (-37.9764, 28.7099) (-38.072, 28.668) (-38.0903, 28.7077) knots 0 0 0 0 1 1 1 1
  spline S1874 degree 3 poles (-38.0903, 28.7077) (-38.1193, 28.7744) (-38.1215, 28.7958) (-38.1279, 28.8464) knots 0 0 0 0 1 1 1 1
  spline S1875 degree 3 poles (-39.9435, 28.2381) (-39.9596, 28.3112) (-39.8855, 28.3918) (-39.8468, 28.2929) knots 0 0 0 0 1 1 1 1
  spline S1876 degree 3 poles (-39.8468, 28.2929) (-39.8113, 28.2037) (-39.8189, 28.164) (-39.8017, 28.1307) knots 0 0 0 0 1 1 1 1
  spline S1877 degree 3 poles (-39.8017, 28.1307) (-39.7856, 28.0963) (-39.8844, 28.0512) (-39.9048, 28.0941) knots 0 0 0 0 1 1 1 1
  spline S1878 degree 3 poles (-39.9048, 28.0941) (-39.9338, 28.1608) (-39.9349, 28.1876) (-39.9435, 28.2381) knots 0 0 0 0 1 1 1 1
  spline S1879 degree 3 poles (-38.433, 28.7744) (-38.448, 28.8485) (-38.375, 28.928) (-38.3363, 28.8292) knots 0 0 0 0 1 1 1 1
  spline S1880 degree 3 poles (-38.3363, 28.8292) (-38.3009, 28.74) (-38.3084, 28.7002) (-38.2912, 28.6669) knots 0 0 0 0 1 1 1 1
  spline S1881 degree 3 poles (-38.2912, 28.6669) (-38.274, 28.6336) (-38.3739, 28.5884) (-38.3943, 28.6314) knots 0 0 0 0 1 1 1 1
  spline S1882 degree 3 poles (-38.3943, 28.6314) (-38.4233, 28.6981) (-38.4244, 28.7249) (-38.433, 28.7744) knots 0 0 0 0 1 1 1 1
  spline S1883 degree 3 poles (-39.1044, 29.1268) (-39.1195, 29.201) (-39.0464, 29.2816) (-39.0078, 29.1816) knots 0 0 0 0 1 1 1 1
  spline S1884 degree 3 poles (-39.0078, 29.1816) (-38.9723, 29.0924) (-38.9798, 29.0527) (-38.9626, 29.0194) knots 0 0 0 0 1 1 1 1
  spline S1885 degree 3 poles (-38.9626, 29.0194) (-38.9454, 28.986) (-39.0454, 28.942) (-39.0658, 28.9839) knots 0 0 0 0 1 1 1 1
  spline S1886 degree 3 poles (-39.0658, 28.9839) (-39.0948, 29.0505) (-39.0958, 29.0774) (-39.1044, 29.1268) knots 0 0 0 0 1 1 1 1
  spline S1887 degree 3 poles (-39.7275, 28.3327) (-39.7447, 28.409) (-39.6695, 28.4939) (-39.6287, 28.3929) knots 0 0 0 0 1 1 1 1
  spline S1888 degree 3 poles (-39.6287, 28.3929) (-39.5911, 28.3005) (-39.5997, 28.2607) (-39.5814, 28.2242) knots 0 0 0 0 1 1 1 1
  spline S1889 degree 3 poles (-39.5814, 28.2242) (-39.5632, 28.1865) (-39.6663, 28.1403) (-39.6878, 28.1844) knots 0 0 0 0 1 1 1 1
  spline S1890 degree 3 poles (-39.6878, 28.1844) (-39.7168, 28.2521) (-39.7179, 28.2833) (-39.7275, 28.3327) knots 0 0 0 0 1 1 1 1
  spline S1891 degree 3 poles (-38.7037, 28.7024) (-38.7209, 28.7787) (-38.6446, 28.8636) (-38.6049, 28.7625) knots 0 0 0 0 1 1 1 1
  spline S1892 degree 3 poles (-38.6049, 28.7625) (-38.5673, 28.6701) (-38.5759, 28.6304) (-38.5576, 28.5927) knots 0 0 0 0 1 1 1 1
  spline S1893 degree 3 poles (-38.5576, 28.5927) (-38.5383, 28.5562) (-38.6414, 28.5089) (-38.664, 28.5541) knots 0 0 0 0 1 1 1 1
  spline S1894 degree 3 poles (-38.664, 28.5541) (-38.693, 28.6207) (-38.6941, 28.6519) (-38.7037, 28.7024) knots 0 0 0 0 1 1 1 1
  spline S1895 degree 3 poles (-39.4289, 28.4101) (-39.4504, 28.4885) (-39.3709, 28.5777) (-39.329, 28.4745) knots 0 0 0 0 1 1 1 1
  spline S1896 degree 3 poles (-39.329, 28.4745) (-39.2892, 28.3789) (-39.2989, 28.3402) (-39.2785, 28.2994) knots 0 0 0 0 1 1 1 1
  spline S1897 degree 3 poles (-39.2785, 28.2994) (-39.2581, 28.2586) (-39.3655, 28.2091) (-39.3881, 28.2564) knots 0 0 0 0 1 1 1 1
  spline S1898 degree 3 poles (-39.3881, 28.2564) (-39.4192, 28.3241) (-39.4203, 28.3596) (-39.4289, 28.4101) knots 0 0 0 0 1 1 1 1
  spline S1899 degree 3 poles (-38.9411, 28.5971) (-38.9605, 28.6766) (-38.8821, 28.7658) (-38.8402, 28.6626) knots 0 0 0 0 1 1 1 1
  spline S1900 degree 3 poles (-38.8402, 28.6626) (-38.8004, 28.567) (-38.8101, 28.5283) (-38.7897, 28.4874) knots 0 0 0 0 1 1 1 1
  spline S1901 degree 3 poles (-38.7897, 28.4874) (-38.7693, 28.4466) (-38.8767, 28.3972) (-38.8993, 28.4444) knots 0 0 0 0 1 1 1 1
  spline S1902 degree 3 poles (-38.8993, 28.4444) (-38.9304, 28.5111) (-38.9315, 28.5455) (-38.9411, 28.5971) knots 0 0 0 0 1 1 1 1
  spline S1903 degree 3 poles (-39.3644, 29.0355) (-39.3838, 29.1139) (-39.3053, 29.2031) (-39.2634, 29.1) knots 0 0 0 0 1 1 1 1
  spline S1904 degree 3 poles (-39.2634, 29.1) (-39.2248, 29.0043) (-39.2344, 28.9656) (-39.213, 28.9248) knots 0 0 0 0 1 1 1 1
  spline S1905 degree 3 poles (-39.213, 28.9248) (-39.1936, 28.884) (-39.3, 28.8345) (-39.3236, 28.8818) knots 0 0 0 0 1 1 1 1
  spline S1906 degree 3 poles (-39.3236, 28.8818) (-39.3537, 28.9495) (-39.3548, 28.985) (-39.3644, 29.0355) knots 0 0 0 0 1 1 1 1
  spline S1907 degree 3 poles (-41.4421, 26.6133) (-41.4432, 26.666) (-41.3927, 26.7111) (-41.3626, 26.6273) knots 0 0 0 0 1 1 1 1
  spline S1908 degree 3 poles (-41.3626, 26.6273) (-41.3401, 26.5628) (-41.339, 26.5177) (-41.3369, 26.5123) knots 0 0 0 0 1 1 1 1
  spline S1909 degree 3 poles (-41.3369, 26.5123) (-41.3347, 26.508) (-41.4045, 26.4844) (-41.4131, 26.5048) knots 0 0 0 0 1 1 1 1
  spline S1910 degree 3 poles (-41.4131, 26.5048) (-41.4378, 26.5714) (-41.4411, 26.5628) (-41.4421, 26.6133) knots 0 0 0 0 1 1 1 1
  spline S1911 degree 3 poles (-41.2402, 26.68) (-41.2445, 26.7369) (-41.1897, 26.7874) (-41.1585, 26.7015) knots 0 0 0 0 1 1 1 1
  spline S1912 degree 3 poles (-41.1585, 26.7015) (-41.1327, 26.6327) (-41.1338, 26.5886) (-41.1284, 26.579) knots 0 0 0 0 1 1 1 1
  spline S1913 degree 3 poles (-41.1284, 26.579) (-41.1252, 26.5693) (-41.1993, 26.5413) (-41.2101, 26.5661) knots 0 0 0 0 1 1 1 1
  spline S1914 degree 3 poles (-41.2101, 26.5661) (-41.2359, 26.6327) (-41.238, 26.6295) (-41.2402, 26.68) knots 0 0 0 0 1 1 1 1
  spline S1915 degree 3 poles (-37.0074, 28.035) (-37.0117, 28.092) (-36.958, 28.1425) (-36.9247, 28.0565) knots 0 0 0 0 1 1 1 1
  spline S1916 degree 3 poles (-36.9247, 28.0565) (-36.901, 27.9878) (-36.901, 27.9437) (-36.8967, 27.934) knots 0 0 0 0 1 1 1 1
  spline S1917 degree 3 poles (-36.8967, 27.934) (-36.8925, 27.9243) (-36.9666, 27.8964) (-36.9773, 27.9211) knots 0 0 0 0 1 1 1 1
  spline S1918 degree 3 poles (-36.9773, 27.9211) (-37.0031, 27.9878) (-37.0053, 27.9845) (-37.0074, 28.035) knots 0 0 0 0 1 1 1 1
  spline S1919 degree 3 poles (-36.7055, 28.0694) (-36.7098, 28.1253) (-36.655, 28.1769) (-36.6239, 28.0909) knots 0 0 0 0 1 1 1 1
  spline S1920 degree 3 poles (-36.6239, 28.0909) (-36.5992, 28.0211) (-36.5992, 27.977) (-36.5949, 27.9673) knots 0 0 0 0 1 1 1 1
  spline S1921 degree 3 poles (-36.5949, 27.9673) (-36.5895, 27.9587) (-36.6647, 27.9308) (-36.6744, 27.9544) knots 0 0 0 0 1 1 1 1
  spline S1922 degree 3 poles (-36.6744, 27.9544) (-36.7012, 28.0211) (-36.7023, 28.0189) (-36.7055, 28.0694) knots 0 0 0 0 1 1 1 1
  spline S1923 degree 3 poles (-36.4874, 28.1694) (-36.4917, 28.2263) (-36.4369, 28.2768) (-36.4058, 28.1908) knots 0 0 0 0 1 1 1 1
  spline S1924 degree 3 poles (-36.4058, 28.1908) (-36.3811, 28.1221) (-36.3811, 28.078) (-36.3768, 28.0683) knots 0 0 0 0 1 1 1 1
  spline S1925 degree 3 poles (-36.3768, 28.0683) (-36.3714, 28.0587) (-36.4466, 28.0318) (-36.4563, 28.0554) knots 0 0 0 0 1 1 1 1
  spline S1926 degree 3 poles (-36.4563, 28.0554) (-36.4831, 28.1221) (-36.4842, 28.1188) (-36.4874, 28.1694) knots 0 0 0 0 1 1 1 1
  spline S1927 degree 3 poles (-40.9716, 26.6972) (-40.978, 26.7573) (-40.92, 26.8132) (-40.8867, 26.7251) knots 0 0 0 0 1 1 1 1
  spline S1928 degree 3 poles (-40.8867, 26.7251) (-40.8599, 26.652) (-40.8609, 26.608) (-40.8545, 26.594) knots 0 0 0 0 1 1 1 1
  spline S1929 degree 3 poles (-40.8545, 26.594) (-40.848, 26.58) (-40.9276, 26.5489) (-40.9394, 26.5768) knots 0 0 0 0 1 1 1 1
  spline S1930 degree 3 poles (-40.9394, 26.5768) (-40.9662, 26.6434) (-40.9684, 26.6467) (-40.9716, 26.6972) knots 0 0 0 0 1 1 1 1
  spline S1931 degree 3 poles (-37.2792, 27.9222) (-37.2856, 27.9834) (-37.2276, 28.0393) (-37.1943, 27.9501) knots 0 0 0 0 1 1 1 1
  spline S1932 degree 3 poles (-37.1943, 27.9501) (-37.1685, 27.8771) (-37.1696, 27.8352) (-37.1632, 27.8201) knots 0 0 0 0 1 1 1 1
  spline S1933 degree 3 poles (-37.1632, 27.8201) (-37.1557, 27.8051) (-37.2352, 27.775) (-37.247, 27.8029) knots 0 0 0 0 1 1 1 1
  spline S1934 degree 3 poles (-37.247, 27.8029) (-37.2661, 27.8399) (-37.2771, 27.8806) (-37.2792, 27.9222) knots 0 0 0 0 1 1 1 1
  spline S1935 degree 3 poles (-40.7707, 26.7982) (-40.7793, 26.8616) (-40.717, 26.9228) (-40.6826, 26.8315) knots 0 0 0 0 1 1 1 1
  spline S1936 degree 3 poles (-40.6826, 26.8315) (-40.6536, 26.7552) (-40.6568, 26.7122) (-40.6472, 26.6929) knots 0 0 0 0 1 1 1 1
  spline S1937 degree 3 poles (-40.6472, 26.6929) (-40.6375, 26.6746) (-40.7224, 26.6402) (-40.7363, 26.6714) knots 0 0 0 0 1 1 1 1
  spline S1938 degree 3 poles (-40.7363, 26.6714) (-40.7563, 26.7109) (-40.768, 26.754) (-40.7707, 26.7982) knots 0 0 0 0 1 1 1 1
  spline S1939 degree 3 poles (-40.5515, 26.882) (-40.5634, 26.9486) (-40.4978, 27.0163) (-40.4613, 26.9228) knots 0 0 0 0 1 1 1 1
  spline S1940 degree 3 poles (-40.4613, 26.9228) (-40.4301, 26.8422) (-40.4344, 26.7992) (-40.4226, 26.7756) knots 0 0 0 0 1 1 1 1
  spline S1941 degree 3 poles (-40.4226, 26.7756) (-40.4108, 26.752) (-40.501, 26.7154) (-40.5161, 26.7498) knots 0 0 0 0 1 1 1 1
  spline S1942 degree 3 poles (-40.5161, 26.7498) (-40.544, 26.8164) (-40.5451, 26.8315) (-40.5515, 26.882) knots 0 0 0 0 1 1 1 1
  spline S1943 degree 3 poles (-37.5703, 27.8309) (-37.5822, 27.8975) (-37.5156, 27.9663) (-37.4801, 27.8728) knots 0 0 0 0 1 1 1 1
  spline S1944 degree 3 poles (-37.4801, 27.8728) (-37.4489, 27.7911) (-37.4532, 27.7492) (-37.4414, 27.7256) knots 0 0 0 0 1 1 1 1
  spline S1945 degree 3 poles (-37.4414, 27.7256) (-37.4296, 27.703) (-37.5188, 27.6643) (-37.5349, 27.6987) knots 0 0 0 0 1 1 1 1
  spline S1946 degree 3 poles (-37.5349, 27.6987) (-37.5551, 27.7401) (-37.5671, 27.7849) (-37.5703, 27.8309) knots 0 0 0 0 1 1 1 1
  spline S1947 degree 3 poles (-40.3098, 26.8841) (-40.3227, 26.9551) (-40.254, 27.0281) (-40.2164, 26.9314) knots 0 0 0 0 1 1 1 1
  spline S1948 degree 3 poles (-40.2164, 26.9314) (-40.183, 26.8476) (-40.1884, 26.8057) (-40.1745, 26.7778) knots 0 0 0 0 1 1 1 1
  spline S1949 degree 3 poles (-40.1745, 26.7778) (-40.1605, 26.7487) (-40.254, 26.7079) (-40.2733, 26.7466) knots 0 0 0 0 1 1 1 1
  spline S1950 degree 3 poles (-40.2733, 26.7466) (-40.3012, 26.8132) (-40.3023, 26.8336) (-40.3098, 26.8841) knots 0 0 0 0 1 1 1 1
  spline S1951 degree 3 poles (-37.7992, 27.7374) (-37.812, 27.8083) (-37.7433, 27.8814) (-37.7057, 27.7847) knots 0 0 0 0 1 1 1 1
  spline S1952 degree 3 poles (-37.7057, 27.7847) (-37.6724, 27.7008) (-37.6778, 27.66) (-37.6638, 27.631) knots 0 0 0 0 1 1 1 1
  spline S1953 degree 3 poles (-37.6638, 27.631) (-37.6498, 27.6031) (-37.7444, 27.5622) (-37.7626, 27.5998) knots 0 0 0 0 1 1 1 1
  spline S1954 degree 3 poles (-37.7626, 27.5998) (-37.7906, 27.6675) (-37.7916, 27.6879) (-37.7992, 27.7374) knots 0 0 0 0 1 1 1 1
  spline S1955 degree 3 poles (-40.125, 26.9894) (-40.1412, 27.0625) (-40.0681, 27.1431) (-40.0294, 27.0432) knots 0 0 0 0 1 1 1 1
  spline S1956 degree 3 poles (-40.0294, 27.0432) (-39.994, 26.9551) (-40.0015, 26.9153) (-39.9843, 26.882) knots 0 0 0 0 1 1 1 1
  spline S1957 degree 3 poles (-39.9843, 26.882) (-39.9671, 26.8498) (-40.067, 26.8046) (-40.0864, 26.8476) knots 0 0 0 0 1 1 1 1
  spline S1958 degree 3 poles (-40.0864, 26.8476) (-40.1164, 26.9132) (-40.1175, 26.939) (-40.125, 26.9894) knots 0 0 0 0 1 1 1 1
  spline S1959 degree 3 poles (-38.0967, 27.617) (-38.1129, 27.6901) (-38.0398, 27.7696) (-38.0001, 27.6707) knots 0 0 0 0 1 1 1 1
  spline S1960 degree 3 poles (-38.0001, 27.6707) (-37.9646, 27.5816) (-37.9721, 27.5418) (-37.9549, 27.5085) knots 0 0 0 0 1 1 1 1
  spline S1961 degree 3 poles (-37.9549, 27.5085) (-37.9388, 27.4752) (-38.0387, 27.4322) (-38.0581, 27.473) knots 0 0 0 0 1 1 1 1
  spline S1962 degree 3 poles (-38.0581, 27.473) (-38.0871, 27.5407) (-38.0882, 27.5665) (-38.0967, 27.617) knots 0 0 0 0 1 1 1 1
  spline S1963 degree 3 poles (-39.879, 27.0894) (-39.8973, 27.1657) (-39.821, 27.2527) (-39.7802, 27.1506) knots 0 0 0 0 1 1 1 1
  spline S1964 degree 3 poles (-39.7802, 27.1506) (-39.7415, 27.0572) (-39.7501, 27.0185) (-39.7318, 26.9798) knots 0 0 0 0 1 1 1 1
  spline S1965 degree 3 poles (-39.7318, 26.9798) (-39.7125, 26.9422) (-39.8167, 26.8949) (-39.8382, 26.94) knots 0 0 0 0 1 1 1 1
  spline S1966 degree 3 poles (-39.8382, 26.94) (-39.8694, 27.0066) (-39.8694, 27.0389) (-39.879, 27.0894) knots 0 0 0 0 1 1 1 1
  spline S1967 degree 3 poles (-38.3685, 27.5429) (-38.3868, 27.6192) (-38.3095, 27.7051) (-38.2686, 27.6041) knots 0 0 0 0 1 1 1 1
  spline S1968 degree 3 poles (-38.2686, 27.6041) (-38.231, 27.5106) (-38.2396, 27.4709) (-38.2203, 27.4343) knots 0 0 0 0 1 1 1 1
  spline S1969 degree 3 poles (-38.2203, 27.4343) (-38.202, 27.3967) (-38.3062, 27.3494) (-38.3277, 27.3946) knots 0 0 0 0 1 1 1 1
  spline S1970 degree 3 poles (-38.3277, 27.3946) (-38.3578, 27.4601) (-38.3589, 27.4924) (-38.3685, 27.5429) knots 0 0 0 0 1 1 1 1
  spline S1971 degree 3 poles (-39.6298, 27.1668) (-39.6513, 27.2463) (-39.5696, 27.3376) (-39.5277, 27.2334) knots 0 0 0 0 1 1 1 1
  spline S1972 degree 3 poles (-39.5277, 27.2334) (-39.488, 27.1377) (-39.4987, 27.0991) (-39.4762, 27.0561) knots 0 0 0 0 1 1 1 1
  spline S1973 degree 3 poles (-39.4762, 27.0561) (-39.4557, 27.0131) (-39.5653, 26.9626) (-39.5879, 27.012) knots 0 0 0 0 1 1 1 1
  spline S1974 degree 3 poles (-39.5879, 27.012) (-39.619, 27.0786) (-39.619, 27.1163) (-39.6298, 27.1668) knots 0 0 0 0 1 1 1 1
  spline S1975 degree 3 poles (-38.5684, 27.4859) (-38.5888, 27.5665) (-38.5082, 27.6568) (-38.4663, 27.5536) knots 0 0 0 0 1 1 1 1
  spline S1976 degree 3 poles (-38.4663, 27.5536) (-38.4266, 27.4558) (-38.4373, 27.4182) (-38.4147, 27.3752) knots 0 0 0 0 1 1 1 1
  spline S1977 degree 3 poles (-38.4147, 27.3752) (-38.3933, 27.3322) (-38.5028, 27.2817) (-38.5265, 27.3312) knots 0 0 0 0 1 1 1 1
  spline S1978 degree 3 poles (-38.5265, 27.3312) (-38.5566, 27.3978) (-38.5576, 27.4354) (-38.5684, 27.4859) knots 0 0 0 0 1 1 1 1
  spline S1979 degree 3 poles (-39.3977, 27.2441) (-39.4214, 27.3279) (-39.3365, 27.4247) (-39.2935, 27.3183) knots 0 0 0 0 1 1 1 1
  spline S1980 degree 3 poles (-39.2935, 27.3183) (-39.2506, 27.2173) (-39.2624, 27.1797) (-39.2387, 27.1324) knots 0 0 0 0 1 1 1 1
  spline S1981 degree 3 poles (-39.2387, 27.1324) (-39.2151, 27.0851) (-39.329, 27.0314) (-39.3548, 27.084) knots 0 0 0 0 1 1 1 1
  spline S1982 degree 3 poles (-39.3548, 27.084) (-39.3848, 27.1506) (-39.3859, 27.1936) (-39.3977, 27.2441) knots 0 0 0 0 1 1 1 1
  spline S1983 degree 3 poles (-38.8273, 27.3613) (-38.8498, 27.4451) (-38.766, 27.5418) (-38.722, 27.4354) knots 0 0 0 0 1 1 1 1
  spline S1984 degree 3 poles (-38.722, 27.4354) (-38.6801, 27.3344) (-38.6919, 27.2979) (-38.6672, 27.2495) knots 0 0 0 0 1 1 1 1
  spline S1985 degree 3 poles (-38.6672, 27.2495) (-38.6446, 27.2022) (-38.7574, 27.1485) (-38.7843, 27.2011) knots 0 0 0 0 1 1 1 1
  spline S1986 degree 3 poles (-38.7843, 27.2011) (-38.8144, 27.2678) (-38.8155, 27.3118) (-38.8273, 27.3613) knots 0 0 0 0 1 1 1 1
  spline S1987 degree 3 poles (-41.5367, 27.0195) (-41.5399, 27.0765) (-41.4862, 27.1227) (-41.4561, 27.0378) knots 0 0 0 0 1 1 1 1
  spline S1988 degree 3 poles (-41.4561, 27.0378) (-41.4325, 26.9712) (-41.4325, 26.9261) (-41.4282, 26.9185) knots 0 0 0 0 1 1 1 1
  spline S1989 degree 3 poles (-41.4282, 26.9185) (-41.4249, 26.911) (-41.4969, 26.8852) (-41.5066, 26.9078) knots 0 0 0 0 1 1 1 1
  spline S1990 degree 3 poles (-41.5066, 26.9078) (-41.5324, 26.9744) (-41.5345, 26.969) (-41.5367, 27.0195) knots 0 0 0 0 1 1 1 1
  spline S1991 degree 3 poles (-37.4597, 28.4573) (-37.4618, 28.5132) (-37.4092, 28.5616) (-37.3791, 28.4767) knots 0 0 0 0 1 1 1 1
  spline S1992 degree 3 poles (-37.3791, 28.4767) (-37.3555, 28.4101) (-37.3555, 28.3639) (-37.3512, 28.3574) knots 0 0 0 0 1 1 1 1
  spline S1993 degree 3 poles (-37.3512, 28.3574) (-37.348, 28.3499) (-37.4199, 28.323) (-37.4296, 28.3467) knots 0 0 0 0 1 1 1 1
  spline S1994 degree 3 poles (-37.4296, 28.3467) (-37.4554, 28.4122) (-37.4575, 28.4079) (-37.4597, 28.4573) knots 0 0 0 0 1 1 1 1
  spline S1995 degree 3 poles (-36.6078, 28.7292) (-36.6099, 28.7851) (-36.5573, 28.8335) (-36.5272, 28.7475) knots 0 0 0 0 1 1 1 1
  spline S1996 degree 3 poles (-36.5272, 28.7475) (-36.5025, 28.6809) (-36.5025, 28.6357) (-36.4993, 28.6293) knots 0 0 0 0 1 1 1 1
  spline S1997 degree 3 poles (-36.4993, 28.6293) (-36.4949, 28.6207) (-36.568, 28.5949) (-36.5777, 28.6175) knots 0 0 0 0 1 1 1 1
  spline S1998 degree 3 poles (-36.5777, 28.6175) (-36.6035, 28.6841) (-36.6045, 28.6787) (-36.6078, 28.7292) knots 0 0 0 0 1 1 1 1
  spline S1999 degree 3 poles (-36.3886, 28.7958) (-36.3918, 28.8507) (-36.3392, 28.899) (-36.3091, 28.8141) knots 0 0 0 0 1 1 1 1
  spline S2000 degree 3 poles (-36.3091, 28.8141) (-36.2844, 28.7464) (-36.2844, 28.7024) (-36.2812, 28.6948) knots 0 0 0 0 1 1 1 1
  spline S2001 degree 3 poles (-36.2812, 28.6948) (-36.2769, 28.6873) (-36.3499, 28.6615) (-36.3585, 28.683) knots 0 0 0 0 1 1 1 1
  spline S2002 degree 3 poles (-36.3585, 28.683) (-36.3843, 28.7507) (-36.3865, 28.7453) (-36.3886, 28.7958) knots 0 0 0 0 1 1 1 1
  spline S2003 degree 3 poles (-36.1834, 28.2564) (-36.1877, 28.3123) (-36.134, 28.3606) (-36.1039, 28.2757) knots 0 0 0 0 1 1 1 1
  spline S2004 degree 3 poles (-36.1039, 28.2757) (-36.0792, 28.2091) (-36.0792, 28.164) (-36.0749, 28.1565) knots 0 0 0 0 1 1 1 1
  spline S2005 degree 3 poles (-36.0749, 28.1565) (-36.0727, 28.1489) (-36.1447, 28.1232) (-36.1544, 28.1457) knots 0 0 0 0 1 1 1 1
  spline S2006 degree 3 poles (-36.1544, 28.1457) (-36.1802, 28.2113) (-36.1823, 28.2059) (-36.1834, 28.2564) knots 0 0 0 0 1 1 1 1
  spline S2007 degree 3 poles (-41.3863, 27.1055) (-41.3938, 27.1657) (-41.3347, 27.2226) (-41.3014, 27.1335) knots 0 0 0 0 1 1 1 1
  spline S2008 degree 3 poles (-41.3014, 27.1335) (-41.2735, 27.0604) (-41.2756, 27.0174) (-41.2681, 27.0023) knots 0 0 0 0 1 1 1 1
  spline S2009 degree 3 poles (-41.2681, 27.0023) (-41.2616, 26.9873) (-41.3422, 26.9561) (-41.353, 26.9841) knots 0 0 0 0 1 1 1 1
  spline S2010 degree 3 poles (-41.353, 26.9841) (-41.3809, 27.0507) (-41.3831, 27.055) (-41.3863, 27.1055) knots 0 0 0 0 1 1 1 1
  spline S2011 degree 3 poles (-37.9678, 28.2628) (-37.9754, 28.323) (-37.9152, 28.3811) (-37.883, 28.2919) knots 0 0 0 0 1 1 1 1
  spline S2012 degree 3 poles (-37.883, 28.2919) (-37.8561, 28.2188) (-37.8583, 28.1747) (-37.8507, 28.1608) knots 0 0 0 0 1 1 1 1
  spline S2013 degree 3 poles (-37.8507, 28.1608) (-37.8421, 28.1446) (-37.9227, 28.1145) (-37.9356, 28.1425) knots 0 0 0 0 1 1 1 1
  spline S2014 degree 3 poles (-37.9356, 28.1425) (-37.955, 28.1798) (-37.966, 28.2209) (-37.9678, 28.2628) knots 0 0 0 0 1 1 1 1
  spline S2015 degree 3 poles (-37.6831, 28.3811) (-37.6896, 28.4412) (-37.6305, 28.4982) (-37.5972, 28.4101) knots 0 0 0 0 1 1 1 1
  spline S2016 degree 3 poles (-37.5972, 28.4101) (-37.5703, 28.3359) (-37.5725, 28.2929) (-37.565, 28.2779) knots 0 0 0 0 1 1 1 1
  spline S2017 degree 3 poles (-37.565, 28.2779) (-37.5574, 28.2628) (-37.6369, 28.2317) (-37.6498, 28.2596) knots 0 0 0 0 1 1 1 1
  spline S2018 degree 3 poles (-37.6498, 28.2596) (-37.6778, 28.3262) (-37.6778, 28.3306) (-37.6831, 28.3811) knots 0 0 0 0 1 1 1 1
  spline S2019 degree 3 poles (-41.1349, 27.1904) (-41.1456, 27.257) (-41.0812, 27.3226) (-41.0457, 27.2302) knots 0 0 0 0 1 1 1 1
  spline S2020 degree 3 poles (-41.0457, 27.2302) (-41.0146, 27.1506) (-41.0189, 27.1087) (-41.0081, 27.0862) knots 0 0 0 0 1 1 1 1